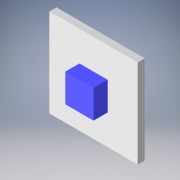
# Autodesk Inventor part: ledstrip
Saved by Autodesk Inventor 2017 (Build 210142000, 142)
## iProperties
Created: 2016-11-07
Part Number: ledstrip
Material: Generic
Document SubType Name: Modeling
Designer: gus
Density: 1 g/cm^3
Appearance: Default
Author: gus
Autodesk Inventor part; units mm, degrees
ref_plane "YZ Plane" through (0, 0, 0) normal (1, 0, 0) x (0, 1, 0)
ref_plane "XZ Plane" through (0, 0, 0) normal (0, 1, 0) x (-1, 0, 0)
ref_plane "XY Plane" through (0, 0, 0) normal (0, 0, 1) x (1, 0, 0)
sketch "Sketch1" plane through (0, 0, 0) normal (0, 0, 1) x (1, 0, 0)
  line L0 (0, 0) -> (15.875, 0)
  line L1 (15.875, 0) -> (15.875, 15.875)
  line L2 (15.875, 15.875) -> (0, 15.875)
  line L3 (0, 15.875) -> (0, 0)
  dimension "d0" = 15.875
  dimension "d1" = 15.875
  constraints: 8 end point, 2 parallel, 1 horizontal, 1 perpendicular
  measures "d0" distance of L2.end L1.end
  measures "d1" distance of L1.end L0.end
extrude "Extrusion1" add sketch "Sketch1" along normal blind 1.27
sketch "Sketch2" plane through (0, 0, 1.27) normal (0, 0, 1) x (1, 0, 0)
  line L0 (0, 0) -> (15.875, 0) projected
  line L1 (15.875, 0) -> (15.875, 15.875) projected
  line L2 (15.875, 15.875) -> (0, 15.875) projected
  line L3 (0, 15.875) -> (0, 0) projected
  line L4 (5.3975, 10.4775) -> (10.4775, 10.4775)
  line L5 (10.4775, 10.4775) -> (10.4775, 5.3975)
  line L6 (10.4775, 5.3975) -> (5.3975, 5.3975)
  line L7 (5.3975, 5.3975) -> (5.3975, 10.4775)
  dimension "d4" = 5.08
  constraints: 8 end point, 3 other
  measures "d4" distance between parallel lines of L5 L7
extrude "Extrusion2" add sketch "Sketch2" along normal blind 2.54 contours L4 L5 L6 L7
body "Solid1"
